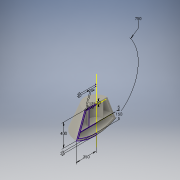
# Autodesk Inventor part: hakoooo
Saved by Autodesk Inventor 2019.3 (Build 233278000, 278)
## iProperties
Created: 2019-01-10
Part Number: hakoooo
Material: 一般
Document SubType Name: Modeling
Designer: masaya
Density: 1 g/cm^3
Appearance: 鋼 - 鋳鋼
Author: masaya
Autodesk Inventor part; units mm, degrees
ref_plane "YZ Plane" through (0, 0, 0) normal (1, 0, 0) x (0, 1, 0)
ref_plane "XZ Plane" through (0, 0, 0) normal (0, 1, 0) x (-1, 0, 0)
ref_plane "XY Plane" through (0, 0, 0) normal (0, 0, 1) x (1, 0, 0)
sketch "スケッチ1" plane through (0, 0, 0) normal (1, 0, 0) x (0, 1, 0)
  line L0 (0, 0) -> (0, 200)
  line L1 (0, 200) -> (-400, 350)
  arc A0 (-400, 350) -> (-486.675, 0) centre (263.325, 0) ccw
  line L2 (-668.2907, 0) -> (453.5942, 0) projected
  line L3 (0, 0) -> (-20, 0)
  line L4 (-20, 0) -> (-20, 180.8)
  line L5 (-20, 180.8) -> (-381.217, 316.2564)
  arc A1 (-381.217, 316.2564) -> (-451.675, 0) centre (293.325, 0) ccw
  line L6 (-451.675, 0) -> (-486.675, 0)
  dimension "d0" = 200
  dimension "d1" = 400
  dimension "d2" = 750
  dimension "d3" = 350
  dimension "d9" = 20
  dimension "d10" = 25
  dimension "d11" = 30
  dimension "d12" = 35
  constraints: 12 end point, 5 point on line, 4 point on circle, 2 centre point, 2 vertical, 1 collinear
  measures "d0" distance of L0.start L0.end
  measures "d1" distance from line of L1.end L0
  measures "d2" radius of A0
  measures "d3" vertical distance of L1.end L6.end
  measures "d9" distance of L0.start L3.end
  measures "d10" distance between parallel lines of L1 L5
  measures "d11" distance of A0.centre A1.centre
  measures "d12" distance of L6.end L6.start
revolve "回転2" add sketch "スケッチ1" angle 180 about axis through (0, -10, 0) along (0, -1, 0) contours L2 L4 L5 A1 A0 L1 L0
sketch "スケッチ2" plane through (0, 263.325, 0) normal (1, 0, 0) x (0, 0, -1)
  line L0 (-284.5531, -560) -> (0, -560)
  line L1 (0, -560) -> (0, -565)
  line L2 (0, -565) -> (-286.4281, -565)
  line L3 (-286.4281, -565) -> (-284.5531, -560)
  line L4 (-316.2564, -644.542) -> (-180.8, -283.325) projected
  arc A0 (-316.2564, -644.542) -> (0, -715) centre (0, 30) ccw projected
  line L5 (0, -906) -> (0, 186) projected
  point P0 (0, -263.325)
  dimension "d14" = 5
  dimension "d15" = 150
  constraints: 8 end point, 3 collinear, 1 horizontal, 1 parallel, 1 perpendicular
  measures "d14" distance of L0.end L1.end
  measures "d15" distance of L1.end A0.end
revolve "回転3" add sketch "スケッチ2" angle 180 about axis through (0, -10, 0) along (0, -1, 0) contours L0 L1 L2 L3
sketch "スケッチ3" plane through (0, 263.325, 0) normal (1, 0, 0) x (0, 0, -1)
  line L0 (-180.8, -283.325) -> (180.8, -283.325) projected
  line L1 (-284.5531, -560) -> (284.5531, -560) projected
  line L2 (-130, -283.325) -> (-130, -560)
  line L3 (-125, -283.325) -> (-125, -560)
  line L4 (0, -847.335) -> (0, -165.9899) projected
  line L5 (-130, -283.325) -> (-125, -283.325)
  line L6 (-130, -560) -> (-125, -560)
  line L7 (-284.5531, -560) -> (284.5531, -560) projected
  point P0 (0, -263.325)
  dimension "d17" = 5
  dimension "d18" = 125
  constraints: 8 end point, 4 point on line, 2 collinear, 2 perpendicular
  measures "d17" distance of L3.start L2.start
  measures "d18" distance from line of L4 L3.start
revolve "回転4" add sketch "スケッチ3" angle 180 about axis through (0, -10, 0) along (0, -1, 0) contours L0 L3 L1 L2
